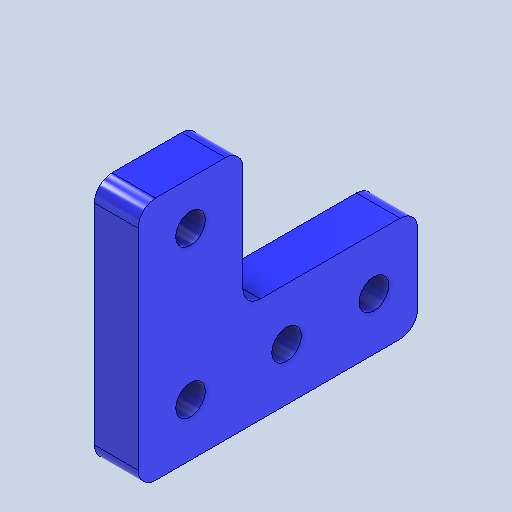
# Autodesk Inventor part: roller-hand-v1-3DP-L-F
Saved by Autodesk Inventor 2025.1 (Build 291241000, 241)
## iProperties
Created: 2024-10-01
Part Number: roller-hand-v1-3DP-L-F
Material: ABS プラスチック
Document SubType Name: Modeling
Designer: haruy
Density: 1.06 g/cm^3
Appearance: 青 - 壁塗料 - 光沢
Author: haruy
Autodesk Inventor part; units mm, degrees
ref_plane "YZ Plane" through (0, 0, 0) normal (1, 0, 0) x (0, 1, 0)
ref_plane "XZ Plane" through (0, 0, 0) normal (0, 1, 0) x (-1, 0, 0)
ref_plane "XY Plane" through (0, 0, 0) normal (0, 0, 1) x (1, 0, 0)
derived "roller-hand-v1-Sketch-Base.ipt"
sketch "スケッチ1" plane through (0, 0, 0) normal (1, 0, 0) x (0, 1, 0)
  circle A0 centre (0, 0) radius 600
  circle A1 centre (0, 0) radius 400
  circle A2 centre (429.926, 0) radius 122.5
  line L0 (-287.7615, 277.8368) -> (287.7615, 277.8368)
  line L1 (287.7615, 277.8368) -> (287.7615, -277.8368)
  line L2 (287.7615, -277.8368) -> (-287.7615, -277.8368)
  line L3 (-287.7615, -277.8368) -> (-287.7615, 277.8368)
  line L4 (-287.7615, 277.8368) -> (287.7615, -277.8368) construction
  line L5 (287.7615, 277.8368) -> (-287.7615, -277.8368) construction
  line L6 (565.0687, 140.5) -> (285.0687, 140.5)
  line L7 (285.0687, 140.5) -> (285.0687, 122.5)
  line L8 (285.0687, 122.5) -> (565.0687, 122.5)
  line L9 (565.0687, 122.5) -> (565.0687, 140.5)
  line L10 (565.0687, -122.5) -> (285.0687, -122.5)
  line L11 (285.0687, -122.5) -> (285.0687, -140.5)
  line L12 (285.0687, -140.5) -> (565.0687, -140.5)
  line L13 (565.0687, -140.5) -> (565.0687, -122.5)
  line L14 (270.0687, 141.5) -> (242.6687, 141.5)
  line L15 (242.6687, 141.5) -> (242.6687, 121.5)
  line L16 (242.6687, 121.5) -> (270.0687, 121.5)
  line L17 (270.0687, 121.5) -> (270.0687, 141.5)
  line L18 (231.8687, 147.5) -> (160.1687, 147.5)
  line L19 (160.1687, 147.5) -> (160.1687, 115.5)
  line L20 (160.1687, 115.5) -> (231.8687, 115.5)
  line L21 (231.8687, 115.5) -> (231.8687, 147.5)
  line L22 (231.8687, 141.5) -> (235.8687, 141.5)
  line L23 (235.8687, 141.5) -> (235.8687, 121.5)
  line L24 (235.8687, 121.5) -> (231.8687, 121.5)
  line L25 (231.8687, 121.5) -> (231.8687, 141.5)
  line L26 (235.8687, 134.5) -> (250.6687, 134.5)
  line L27 (250.6687, 134.5) -> (250.6687, 128.5)
  line L28 (250.6687, 128.5) -> (235.8687, 128.5)
  line L29 (235.8687, 128.5) -> (235.8687, 134.5)
  line L30 (300.0687, 136.5) -> (262.0687, 136.5)
  line L31 (262.0687, 136.5) -> (262.0687, 126.5)
  line L32 (262.0687, 126.5) -> (300.0687, 126.5)
  line L33 (300.0687, 126.5) -> (300.0687, 136.5)
  line L34 (280.0687, 145.0404) -> (275.0687, 145.0404)
  line L35 (275.0687, 145.0404) -> (275.0687, 91.5358)
  line L36 (275.0687, 91.5358) -> (280.0687, 91.5358)
  line L37 (280.0687, 91.5358) -> (280.0687, 145.0404)
  line L38 (275.0687, 145.5) -> (263.0687, 145.5)
  line L39 (263.0687, 145.5) -> (263.0687, -145.5)
  line L40 (263.0687, -145.5) -> (275.0687, -145.5)
  line L41 (275.0687, -145.5) -> (275.0687, 145.5)
  line L42 (565.0687, 157.5) -> (263.0687, 157.5)
  line L43 (263.0687, 157.5) -> (263.0687, 145.5)
  line L44 (263.0687, 145.5) -> (565.0687, 145.5)
  line L45 (565.0687, 145.5) -> (565.0687, 157.5)
  line L46 (575.0687, 157.5) -> (570.0687, 157.5)
  line L47 (570.0687, 157.5) -> (570.0687, 122.5)
  line L48 (570.0687, 122.5) -> (575.0687, 122.5)
  line L49 (575.0687, 122.5) -> (575.0687, 157.5)
  line L50 (565.0687, -145.5) -> (263.0687, -145.5)
  line L51 (263.0687, -145.5) -> (263.0687, -157.5)
  line L52 (263.0687, -157.5) -> (565.0687, -157.5)
  line L53 (565.0687, -157.5) -> (565.0687, -145.5)
  circle A3 centre (269.0687, 140.5) radius 1.7
  circle A4 centre (269.0687, 130.5) radius 1.7
  circle A5 centre (269.0687, 151.5) radius 1.7
  circle A6 centre (286.0687, 151.5) radius 1.7
  circle A7 centre (555.0687, 151.5) radius 1.5
  circle A8 centre (545.0687, 151.5) radius 1.5
  line L54 (0, 0) -> (429.926, 0)
  circle A9 centre (555.0687, -151.5) radius 1.5
  circle A10 centre (545.0687, -151.5) radius 1.5
  circle A11 centre (269.0687, -130.5) radius 1.7
  circle A12 centre (269.0687, -140.5) radius 1.7
  circle A13 centre (269.0687, -151.5) radius 1.7
  circle A14 centre (286.0687, -151.5) radius 1.7
  line L55 (291.0687, 157.5) -> (291.0687, 145.5)
  line L56 (275.0687, 125.5) -> (263.0687, 125.5)
  dimension "d1" = 5
  dimension "d2" = 5
  measures "d1" distance from line of L55 A6.centre
  measures "d2" distance from line of L56 A4.centre
sketch "スケッチ2" plane through (0, 0, 0) normal (0, 1, 0) x (-1, 0, 0)
  circle A0 centre (0, 0) radius 9
  line L0 (33, 14) -> (21, 14)
  line L1 (21, 14) -> (21, -141.0479)
  line L2 (21, -141.0479) -> (33, -141.0479)
  line L3 (33, -141.0479) -> (33, 14)
  line L4 (33, 26) -> (21, 26)
  line L5 (21, 26) -> (21, 14)
  line L6 (21, 14) -> (33, 14)
  line L7 (33, 14) -> (33, 26)
  circle A1 centre (0, 0) radius 16
  circle A2 centre (0, 0) radius 21
  circle A3 centre (14.8492, 14.8492) radius 1.7
  circle A4 centre (-14.8492, 14.8492) radius 1.7
  circle A5 centre (-14.8492, -14.8492) radius 1.7
  circle A6 centre (14.8492, -14.8492) radius 1.7
  circle A7 centre (14.8492, 14.8492) radius 4.7
  circle A8 centre (14.8492, -14.8492) radius 4.7
  circle A9 centre (-14.8492, 14.8492) radius 4.7
  circle A10 centre (-14.8492, -14.8492) radius 4.7
  circle A11 centre (27, 4) radius 1.7
  circle A12 centre (27, -6) radius 1.7
  line L8 (21, 14) -> (18.7936, 17.4051)
  line L9 (14.8492, 19.5492) -> (-14.8492, 19.5492)
  line L10 (-19.5492, 14.8492) -> (-19.5492, -14.8492)
  line L11 (-14.8492, -19.5492) -> (14.8492, -19.5492)
  line L12 (33, -19.5492) -> (21, -19.5492)
  line L13 (21, -19.5492) -> (14.8492, -19.5492)
  circle A13 centre (0, 0) radius 7.55
  circle A14 centre (14.8492, 14.8492) radius 3
  circle A15 centre (14.8492, -14.8492) radius 3
  circle A16 centre (-14.8492, 14.8492) radius 3
  circle A17 centre (-14.8492, -14.8492) radius 3
  point P0 (0, 21)
extrude "押し出し1" add sketch "スケッチ1" against normal blind 5 contours L42 L55 L44 L1 A6 | L1 A6 L44 L38 L43 L42 | L38 L41 L35 L30 L17 A3 L14 L39 | L14 A3 L17 L30 L39 | L30 L17 A4 L32 L39 | L35 L32 L17 A4 L30 | L32 L17 L56 L39 | L35 L56 L17 L32
fillet "フィレット1" radius 2 6 edges at (-2.5, 263.0687, 125.5) (-2.5, 263.0687, 157.5) (-2.5, 275.0687, 145.5) (-2.5, 275.0687, 125.5) (-2.5, 291.0687, 145.5) (-2.5, 291.0687, 157.5)
